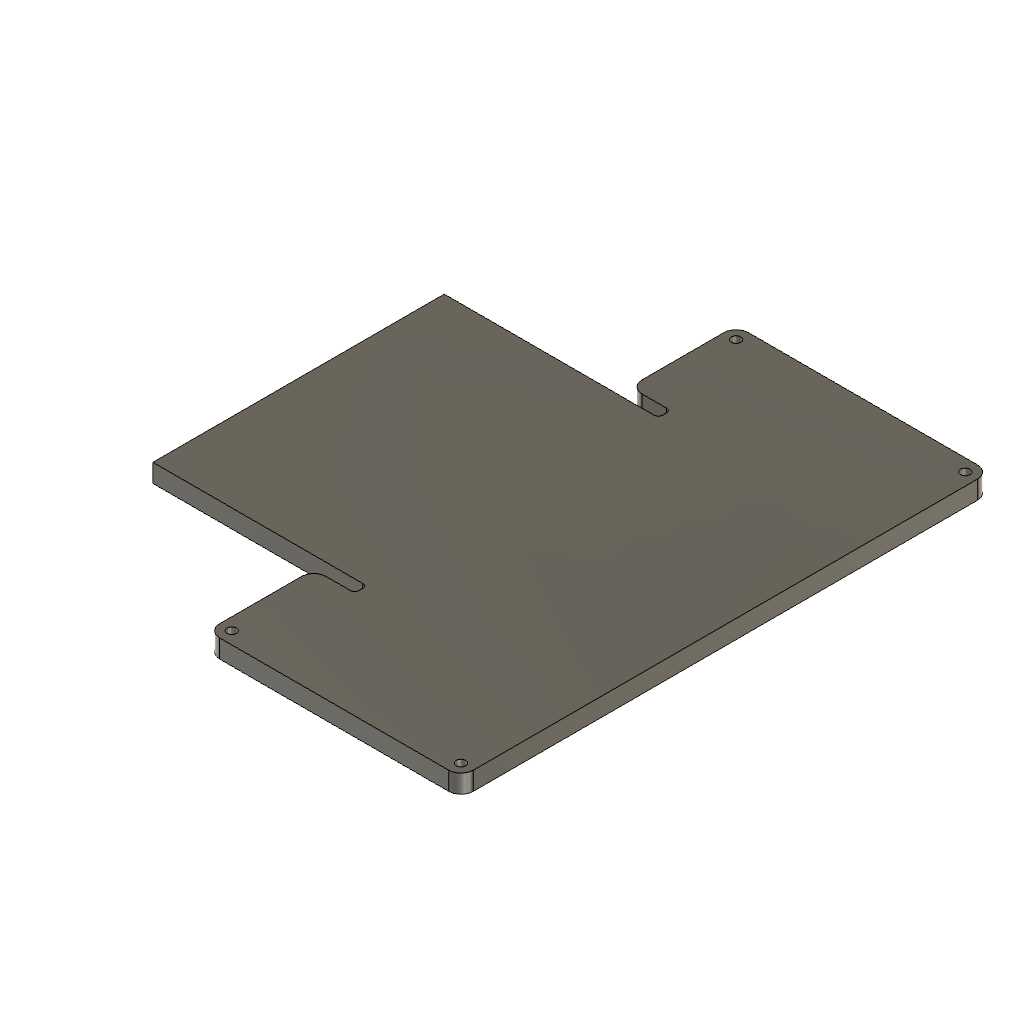
BottomCover_HD1370A (Autodesk Fusion 360 design; units mm, degrees)
part number: 2026-09-25-20-10-25-456
Autodesk Fusion 360 part; units mm, degrees
sketch "Exact underside rim - R3 desk, R1 shoulders, square chair" plane through (0, 0, 0) normal (0, 0, 1) x (1, 0, 0)
  line L0 (-75.3, 35.6) -> (-24, 35.6)
  arc A0 (-24, 35.6) -> (-23, 36.6) centre (-24, 36.6) ccw
  line L1 (-23, 36.6) -> (-23, 37.6)
  arc A1 (-23, 37.6) -> (-24, 38.6) centre (-24, 37.6) ccw
  line L2 (-24, 38.6) -> (-30, 38.6)
  arc A2 (-33, 41.6) -> (-30, 38.6) centre (-30, 41.6) ccw
  line L3 (-33, 41.6) -> (-33, 61.6)
  arc A3 (-30, 64.6) -> (-33, 61.6) centre (-30, 61.6) ccw
  line L4 (-30, 64.6) -> (26, 64.6)
  arc A4 (29, 61.6) -> (26, 64.6) centre (26, 61.6) ccw
  line L5 (29, 61.6) -> (29, -61.6)
  arc A5 (26, -64.6) -> (29, -61.6) centre (26, -61.6) ccw
  line L6 (26, -64.6) -> (-30, -64.6)
  arc A6 (-33, -61.6) -> (-30, -64.6) centre (-30, -61.6) ccw
  line L7 (-33, -61.6) -> (-33, -41.6)
  arc A7 (-30, -38.6) -> (-33, -41.6) centre (-30, -41.6) ccw
  line L8 (-30, -38.6) -> (-24, -38.6)
  arc A8 (-24, -38.6) -> (-23, -37.6) centre (-24, -37.6) ccw
  line L9 (-23, -37.6) -> (-23, -36.6)
  arc A9 (-23, -36.6) -> (-24, -35.6) centre (-24, -36.6) ccw
  line L10 (-24, -35.6) -> (-75.3, -35.6)
  line L11 (-75.3, -35.6) -> (-75.3, 35.6)
extrude "Plate - exact flush rim and flat floor" add sketch "Exact underside rim - R3 desk, R1 shoulders, square chair" along normal blind 4.5
sketch "M2 through holes" plane through (0, 0, 0) normal (0, 0, 1) x (1, 0, 0)
  circle A0 centre (-30, -61.6) radius 1.15
  circle A1 centre (26, -61.6) radius 1.15
  circle A2 centre (-30, 61.6) radius 1.15
  circle A3 centre (26, 61.6) radius 1.15
  dimension "d8" = 2.3
  dimension "d9" = 2.3
  dimension "d10" = 2.3
  dimension "d11" = 2.3
  measures "d8" diameter of A0
  measures "d9" diameter of A1
  measures "d10" diameter of A2
  measures "d11" diameter of A3
extrude "M2 through holes (1)" cut sketch "M2 through holes" along normal blind 4.5
sketch "Recessed M2 heads on floor side" plane through (0, 0, 0) normal (0, 0, 1) x (1, 0, 0)
  circle A0 centre (-30, -61.6) radius 2.15
  circle A1 centre (26, -61.6) radius 2.15
  circle A2 centre (-30, 61.6) radius 2.15
  circle A3 centre (26, 61.6) radius 2.15
  dimension "d14" = 4.3
  dimension "d15" = 4.3
  dimension "d16" = 4.3
  dimension "d17" = 4.3
  measures "d14" diameter of A0
  measures "d15" diameter of A1
  measures "d16" diameter of A2
  measures "d17" diameter of A3
extrude "Recessed M2 heads on floor side (1)" cut sketch "Recessed M2 heads on floor side" along normal blind 2.3
equation "plate_thickness = 4.5 mm" comment "Overall plate thickness"
equation "clearance = 0.3 mm" comment "Original robot CAD clearance"
equation "screw_diameter = 2 mm" comment "M2 nominal shaft diameter"
equation "screw_head_diameter = 4 mm" comment "Original CAD head envelope"
equation "screw_head_height = 2 mm" comment "Original CAD head height envelope"
equation "d6 = plate_thickness"
equation "d8 = screw_diameter + clearance"
equation "d9 = screw_diameter + clearance"
equation "d10 = screw_diameter + clearance"
equation "d11 = screw_diameter + clearance"
equation "d12 = plate_thickness"
equation "d14 = screw_head_diameter + clearance"
equation "d15 = screw_head_diameter + clearance"
equation "d16 = screw_head_diameter + clearance"
equation "d17 = screw_head_diameter + clearance"
equation "d18 = screw_head_height + clearance"
named bodies: "BottomCover"
